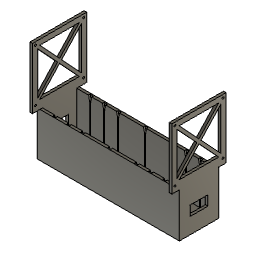
20220624_chipholder (Autodesk Fusion 360 design; units mm, degrees)
Autodesk Fusion 360 part; units mm, degrees
note: some values were not read from the file. Chosen so that the rebuilt part matches the saved one: a direction; which face or edge a step refers to. Set by a fixed rule: which sketch regions a step uses.
sketch "Sketch1" plane through (0, 0, 0) normal (0, 1, 0) x (1, 0, 0)
  line L0 (0, 0) -> (250, 0) construction
  line L1 (0, -70) -> (262.6, -70) construction
  line L2 (0, -80) -> (256.8, -80) construction
  line L3 (25, 0) -> (25, -70)
  line L4 (26.8, -70) -> (26.8, 0)
  line L5 (25, -70) -> (23, -80)
  line L6 (26.8, -70) -> (28.8, -80)
  line L7 (51.8, 0) -> (51.8, -70)
  line L8 (53.6, -70) -> (53.6, 0)
  line L9 (51.8, -70) -> (49.8, -80)
  line L10 (53.6, -70) -> (55.6, -80)
  line L11 (78.6, -70) -> (78.6, 0)
  line L12 (210.8, 0) -> (210.8, -70)
  line L13 (80.4, -70) -> (80.4, 0)
  line L14 (130.4, 0) -> (130.4, -70)
  line L15 (132.2, -70) -> (132.2, 0)
  line L16 (182.2, 0) -> (182.2, -70)
  line L17 (209, -70) -> (209, 0)
  line L18 (237.6, 0) -> (237.6, -70)
  line L19 (235.8, -70) -> (235.8, 0)
  line L20 (184, 0) -> (184, -70)
  line L21 (78.6, -70) -> (76.6, -80)
  line L22 (80.4, -70) -> (82.4, -80)
  line L23 (130.4, -70) -> (128.4, -80)
  line L24 (182.2, -70) -> (180.2, -80)
  line L25 (235.8, -70) -> (233.8, -80)
  line L26 (237.6, -70) -> (239.6, -80)
  line L27 (132.2, -70) -> (134.2, -80)
  line L28 (184, -70) -> (186, -80)
  line L29 (209, -70) -> (207, -80)
  line L30 (210.8, -70) -> (212.8, -80)
  line L31 (0, -80) -> (262.6, -80)
  line L32 (262.6, -80) -> (262.6, 0)
  line L33 (262.6, 0) -> (0, 0)
  line L34 (0, 0) -> (0, -80)
  dimension "d2" = 70
  dimension "d3" = 80
  dimension "d5" = 1.8
  dimension "d6" = 2
  dimension "d7" = 2
  dimension "d8" = 25
  dimension "d9" = 1.8
  dimension "d10" = 2
  dimension "d11" = 2
  dimension "d12" = 25
  dimension "d13" = 1.8
  dimension "d14" = 50
  dimension "d15" = 1.8
  dimension "d16" = 50
  dimension "d17" = 1.8
  dimension "d18" = 25
  dimension "d19" = 1.8
  dimension "d20" = 25
  dimension "d21" = 1.8
  dimension "d22" = 2
  dimension "d23" = 2
  dimension "d24" = 2
  dimension "d25" = 2
  dimension "d26" = 2
  dimension "d27" = 2
  dimension "d28" = 2
  dimension "d29" = 2
  dimension "d30" = 2
  dimension "d31" = 2
  dimension "d32" = 25
  dimension "d33" = 80
  constraint coincident L0.start L33.end
  constraint horizontal L0
  constraint horizontal L1
  constraint parallel L1 L2
  constraint coincident L0 L3.start
  constraint coincident L1 L3.end
  constraint perpendicular L1 L3
  constraint coincident L1 L4.start
  constraint coincident L0 L4.end
  constraint perpendicular L0 L4
  constraint coincident L2 L5.end
  constraint coincident L2 L6.end
  constraint coincident L0 L7.start
  constraint coincident L1 L7.end
  constraint perpendicular L1 L7
  constraint coincident L1 L8.start
  constraint coincident L0 L8.end
  constraint perpendicular L0 L8
  constraint coincident L2 L9.end
  constraint coincident L2 L10.end
  constraint coincident L1 L11.start
  constraint coincident L0 L11.end
  constraint perpendicular L0 L11
  constraint coincident L0 L12.start
  constraint coincident L1 L12.end
  constraint coincident L1 L13.start
  constraint coincident L0 L13.end
  constraint perpendicular L0 L13
  constraint coincident L0 L14.start
  constraint coincident L1 L14.end
  constraint perpendicular L1 L14
  constraint coincident L1 L15.start
  constraint coincident L0 L15.end
  constraint perpendicular L0 L15
  constraint coincident L0 L16.start
  constraint coincident L1 L16.end
  constraint perpendicular L1 L16
  constraint coincident L1 L17.start
  constraint coincident L0 L17.end
  constraint perpendicular L0 L17
  constraint coincident L0 L18.start
  constraint coincident L1 L18.end
  constraint perpendicular L1 L18
  constraint coincident L1 L19.start
  constraint coincident L0 L19.end
  constraint perpendicular L0 L19
  constraint coincident L0 L20.start
  constraint perpendicular L0 L20
  constraint coincident L2 L21.end
  constraint coincident L2 L22.end
  constraint midpoint L2 L23.end
  constraint coincident L2 L24.end
  constraint coincident L2 L25.end
  constraint coincident L2 L26.end
  constraint coincident L1 L20.end
  constraint coincident L2 L27.end
  constraint coincident L2 L28.end
  constraint coincident L2 L29.end
  constraint coincident L2 L30.end
  constraint horizontal L31
  constraint vertical L32
  constraint horizontal L33
  constraint vertical L34
  constraint coincident L1.end L32
  measures "d2" distance of L0 L1
  measures "d3" distance of L0 L2
  measures "d5" distance of L3 L4
  measures "d6" distance of L3 L5.end
  measures "d7" distance of L4 L6.end
  measures "d8" distance of L4 L7
  measures "d9" distance of L7 L8
  measures "d10" distance of L7 L9.end
  measures "d11" distance of L8 L10.end
  measures "d12" distance of L8 L11
  measures "d13" distance of L11 L13
  measures "d14" distance of L13 L14
  measures "d15" distance of L14 L15
  measures "d16" distance of L15 L16
  measures "d17" distance of L16 L20
  measures "d18" distance of L17 L20
  measures "d19" distance of L12 L17
  measures "d20" distance of L12 L19
  measures "d21" distance of L18 L19
  measures "d22" distance of L11 L21.end
  measures "d23" distance of L13 L22.end
  measures "d24" distance of L14 L23.end
  measures "d25" distance of L15 L27.end
  measures "d26" distance of L16 L24.end
  measures "d27" distance of L20 L28.end
  measures "d28" distance of L17 L29.end
  measures "d29" distance of L12 L30.end
  measures "d30" distance of L19 L25.end
  measures "d31" distance of L18 L26.end
  measures "d32" distance of L18 L32
  measures "d33" distance of L31 L33
extrude "Extrude1" add sketch "Sketch1" along normal blind 5 makes body 1
extrude "Extrude2" cut sketch "Sketch1" along normal blind 3 contours L3 L4 L5 L6 L31 L33 | L7 L8 L9 L10 L31 L33 | L11 L13 L21 L22 L31 L33 | L14 L15 L23 L27 L31 L33 | L16 L20 L24 L28 L31 L33 | L12 L17 L29 L30 L31 L33 | L18 L19 L25 L26 L31 L33 bodies 1
copy_body "CopyPasteBodies1" bodies 1 makes body 2
move_body "Move1" bodies 2 to x (1, 0, 0) y (0, 1, 0) z (0, 0, 1) at (0, -71.4, 0)
move_body "Move2" bodies 2 to x (-1, 0, 0) y (0, -1, 0) z (0, 0, 1) at (260.8, -142.8, 0)
move_body "Move3" bodies 2 to x (1, 0, 0) y (0, 1, 0) z (0, 0, 1) at (0, 6, 0)
sketch "Sketch1 (2)" plane through (0, 0, 0) normal (0, 0, 1) x (1, 0, 0) in component "carrier"
  line L0 (-40.0005, -7.3553) -> (29.9995, -7.3553)
  line L1 (29.9995, -7.3553) -> (29.9995, 62.6447)
  line L2 (-40.0005, 62.6447) -> (-40.0005, -7.3553)
  line L3 (-40.0005, 62.6447) -> (-31.0005, 62.6447)
  line L4 (29.9995, 62.6447) -> (20.9995, 62.6447)
  line L5 (-31.0005, 62.6447) -> (-31.0005, 79.6447)
  line L6 (20.9995, 62.6447) -> (20.9995, 79.6447)
  line L7 (20.9995, 79.6447) -> (44.9995, 79.6447)
  line L8 (44.9995, 79.6447) -> (44.9995, 187.4447)
  line L9 (44.9995, 187.4447) -> (-55.0005, 187.4447)
  line L10 (-55.0005, 187.4447) -> (-55.0005, 79.6447)
  line L11 (-55.0005, 79.6447) -> (-31.0005, 79.6447)
  circle A0 centre (-51.1505, 83.4947) radius 1.95
  circle A1 centre (41.1495, 83.4947) radius 1.95
  circle A2 centre (41.1495, 183.5947) radius 1.95
  circle A3 centre (-51.1505, 183.5947) radius 1.95
  line L12 (75.2881, -7.3553) -> (70.2881, -7.3553)
  dimension "d18_1" = 70
  dimension "d23_1" = 9
  dimension "d24_1_1" = 9
  dimension "d25_1_1" = 70
  dimension "d26_1_1" = 52
  dimension "d27_1_1" = 17
  dimension "d28_1" = 17
  dimension "d29_1_1" = 70
  dimension "d47" = 107.8
  dimension "d48" = 100
  dimension "d49" = 3.9
  dimension "d50" = 3.85
  dimension "d51" = 3.85
  dimension "d52" = 3.9
  dimension "d53" = 3.9
  dimension "d54" = 3.9
  dimension "d55" = 3.85
  dimension "d56" = 3.85
  dimension "d57" = 3.85
  dimension "d58" = 3.85
  dimension "d59" = 3.85
  dimension "d60" = 3.85
  constraint horizontal L0
  constraint vertical L1
  constraint vertical L2
  constraint perpendicular L1 L4
  constraint perpendicular L6 L7
  constraint perpendicular L7 L8
  constraint perpendicular L8 L9
  constraint perpendicular L9 L10
  constraint perpendicular L5 L11
  constraint equal L7 L11
  constraint collinear L0 L12
  constraint parallel L0 L9
  measures "d18_1" distance of L0.start L0.end
  measures "d23_1" distance of L2.start L3.end
  measures "d24_1_1" distance of L1.end L4.end
  measures "d25_1_1" distance of L0.end L1.end
  measures "d26_1_1" distance of L5.end L6.end
  measures "d27_1_1" distance of L4.end L6.end
  measures "d28_1" distance of L3.end L5.end
  measures "d29_1_1" distance of L0.start L2.start
  measures "d47" distance of L9 L11
  measures "d48" distance of L8 L10
  measures "d49" diameter of A0
  measures "d50" distance of L11 A0.centre
  measures "d51" distance of L10 A0.centre
  measures "d52" diameter of A1
  measures "d53" diameter of A2
  measures "d54" diameter of A3
  measures "d55" distance of L7 A1.centre
  measures "d56" distance of L8 A1.centre
  measures "d57" distance of L9 A3.centre
  measures "d58" distance of L10 A3.centre
  measures "d59" distance of L9 A2.centre
  measures "d60" distance of L8 A2.centre
extrude "Extrude1'" add sketch "Sketch1 (2)" along normal blind 1.6 separate body contours L0 L1 L2 L3 L4 L5 L6 L7 L8 L9 L10 L11 | A0 | A1 | A2 | A3 makes body 3 in component "carrier"
sketch "Sketch2" plane through (0, 0, 1.7) normal (0, 0, 1) x (-1, 0, 0) in component "carrier"
  line L0 (-200, -70) -> (-200, 0)
  line L1 (-200, 0) -> (-270, 0)
  line L2 (-270, 0) -> (-270, -70)
  line L3 (-270, -70) -> (-261, -70)
  line L4 (-261, -70) -> (-261, -83.4)
  line L5 (-261, -83.4) -> (-209, -83.4)
  line L6 (-209, -83.4) -> (-209, -70)
  line L7 (-209, -70) -> (-200, -70)
  line L8 (-207, -21) -> (-207, -49)
  line L9 (-270, 0) -> (-268.2738, 0)
  line L10 (-268.2738, -21) -> (-270, -21)
  line L11 (-270, -21) -> (-268.2738, -21)
  line L12 (-263, -21) -> (-263, -49)
  line L13 (-207, -49) -> (-263, -49)
  line L14 (-207, -21) -> (-263, -21)
  dimension "d38_1" = 7
  dimension "d39_1_1" = 7
  dimension "d40_1_1" = 21
  dimension "d41_1_1" = 21
  constraint horizontal L9
  constraint horizontal L10
  constraint coincident L1.end L2.start
  constraint perpendicular L2 L11
  constraint perpendicular L11 L12
  measures "d38_1" distance of L0 L8
  measures "d39_1_1" distance of L2 L12
  measures "d40_1_1" distance of L1 L14
  measures "d41_1_1" distance of L3 L13
extrude "Extrude2'" [suppressed] in component "carrier"
sketch "Sketch3" plane through (0, 0, 6.2) normal (0, 0, 1) x (-1, 0, 0) in component "carrier"
  line L0 (-207, -49) -> (-207, -21)
  line L1 (-207, -21) -> (-263, -21)
  line L2 (-263, -21) -> (-263, -49)
  line L3 (-263, -49) -> (-207, -49)
  circle A0 centre (-209.7, -35) radius 2.7
  line L4 (-270, 0) -> (-235, 0) construction
  line L5 (-235, 0) -> (-235, -95) construction
  circle A1 centre (-260.3, -35) radius 2.7
  dimension "d44_1_1" = 5.4
  dimension "d45_1" = 14
  dimension "d47_1" = 2.7
  dimension "d48_1" = 35
  dimension "d49_1" = 14
  dimension "d50_1" = 2.7
  constraint horizontal L4
  constraint perpendicular L1 L5
  constraint symmetric A0 L5 A1
  measures "d44_1_1" diameter of A0
  measures "d45_1" distance of L1 A0.centre
  measures "d47_1" distance of L0 A0.centre
  measures "d48_1" distance of L4.start L4.end
  measures "d49_1" distance of L3 A1.centre
  measures "d50_1" distance of L2 A1.centre
extrude "Extrude4" [suppressed] in component "carrier"
extrude "Extrude3" [suppressed] in component "carrier"
sketch "Sketch5" plane through (0, 0, 0) normal (0, 0, -1) x (1, 0, 0) in component "carrier"
  line L0 (200, 0) -> (200, -70)
  line L1 (200, -70) -> (209, -70)
  line L2 (209, -70) -> (209, -83.4)
  line L3 (209, -83.4) -> (261, -83.4)
  line L4 (261, -83.4) -> (261, -70)
  line L5 (261, -70) -> (270, -70)
  line L6 (270, -70) -> (270, 0)
  line L7 (270, 0) -> (200, 0)
  line L8 (206.7865, -21) -> (206.7865, -49)
  line L9 (263, -21) -> (263, -49)
  line L10 (206.7865, -21) -> (263, -21)
  line L11 (206.7865, -49) -> (263, -49)
  dimension "d61_1" = 28
  dimension "d62_1" = 28
  constraint perpendicular L9 L10
  constraint perpendicular L9 L11
  measures "d61_1" distance of L8.start L8.end
  measures "d62_1" distance of L9.start L9.end
extrude "Extrude6" [suppressed] in component "carrier"
sketch "Sketch7" plane through (0, 0, -4.5) normal (0, 0, -1) x (1, 0, 0) in component "carrier"
  line L0 (206.7865, -21) -> (206.7865, -49)
  line L1 (206.7865, -49) -> (263, -49)
  line L2 (263, -49) -> (263, -21)
  line L3 (263, -21) -> (206.7865, -21)
  circle A0 centre (209.4865, -35) radius 2.7
  line L4 (206.7865, -21) -> (206.7865, -49)
  line L5 (206.7865, -21) -> (263, -21)
  line L6 (235, 0) -> (235, -95)
  circle A1 centre (260.5135, -35) radius 2.7
  dimension "d73_1" = 5.4
  dimension "d74_1" = 2.7
  dimension "d75_1" = 14
  constraint symmetric A0 L6 A1
  measures "d73_1" diameter of A0
  measures "d74_1" distance of A0.centre L4
  measures "d75_1" distance of A0.centre L5
extrude "Extrude8" [suppressed] in component "carrier"
extrude "Extrude7" [suppressed] in component "carrier"
sketch "Sketch8" plane through (0, 0, -6.8) normal (0, 0, -1) x (1, 0, 0) in component "carrier"
  circle A0 centre (209.4865, -35) radius 2.7
  circle A1 centre (209.4865, -35) radius 1.5
  dimension "d80_1" = 3
  constraint concentric A0 A1
  measures "d80_1" diameter of A1
extrude "Extrude9" [suppressed] in component "carrier"
sketch "Sketch10" plane through (0, 0, -6.8) normal (0, 0, -1) x (1, 0, 0) in component "carrier"
  line L0 (263, -36.0522) -> (263, -33.9478)
  arc A0 (263, -33.9478) -> (263, -36.0522) centre (260.5135, -35) ccw
  circle A1 centre (260.5135, -35) radius 1.5
  dimension "d84_1" = 3
  constraint concentric A0 A1
  measures "d84_1" diameter of A1
extrude "Extrude10" [suppressed] in component "carrier"
sketch "Sketch1 (3)" plane through (0, 0, 1.6) normal (0, 0, 1) x (-1, 0, 0) in component "alpide sensor"
  circle A0 centre (-65, -5) radius 1.5
  circle A1 centre (-5, -5) radius 1.5
  circle A2 centre (-65, -65) radius 1.5
  circle A3 centre (-5, -65) radius 1.5
  line L0 (0, -70) -> (0, 0)
  line L1 (0, 0) -> (-70, 0)
  line L2 (-70, 0) -> (-70, -70)
  line L3 (-70, -70) -> (-61, -70)
  line L4 (-61, -70) -> (-61, -83.5)
  line L5 (-61, -83.5) -> (-9, -83.5)
  line L6 (-9, -83.5) -> (-9, -70)
  line L7 (-9, -70) -> (0, -70)
  line L8 (-20, -42.5) -> (-50, -42.5)
  line L9 (-50, -42.5) -> (-50, -27.5)
  line L10 (-50, -27.5) -> (-20, -27.5)
  line L11 (-20, -27.5) -> (-20, -42.5)
  dimension "d58_1" = 30
  dimension "d59_1" = 15
  dimension "d60_1" = 41
  dimension "d63_1" = 20
  constraint horizontal L8
  constraint vertical L9
  constraint horizontal L10
  constraint vertical L11
  measures "d58_1" distance of L8.start L8.end
  measures "d59_1" distance of L8.start L10.end
  measures "d60_1" distance of L5 L8
  measures "d63_1" distance of L2 L9
extrude "Extrude1''" add sketch "Sketch1 (3)" along normal blind -1.8 and the other way blind -0.1 separate body contours L8 L9 L10 L11 makes body 4 in component "alpide sensor"
move_body "Move4" bodies 2 to x (1, 0, 0) y (0, 1, 0) z (0, 0, 1) at (1.7002, -8.1148, 0)
move_body "Move5" bodies 2 to x (1, 0, 0) y (0, 1, 0) z (0, 0, 1) at (0.0998, 78.5148, 0)
move_body "Move6" bodies 2 to x (1, 0, 0) y (0, 1, 0) z (0, 0, 1) at (0, -71.4, 0)
move_body "Move7" bodies 2 to x (1, 0, 0) y (0, 1, 0) z (0, 0, 1) at (0, 1, 0)
sketch "Sketch2 (2)" plane through (0, 0, 0) normal (0, 0, -1) x (1, 0, 0)
  line L0 (182.2, -3) -> (182.2, 0)
  line L1 (182.2, 0) -> (132.2, 0)
  line L2 (132.2, 0) -> (132.2, -3)
  line L3 (132.2, -3) -> (130.4, -3)
  line L4 (130.4, -3) -> (130.4, 0)
  line L5 (130.4, 0) -> (80.4, 0)
  line L6 (80.4, 0) -> (80.4, -3)
  line L7 (80.4, -3) -> (78.6, -3)
  line L8 (78.6, -3) -> (78.6, 0)
  line L9 (78.6, 0) -> (53.6, 0)
  line L10 (53.6, 0) -> (53.6, -3)
  line L11 (53.6, -3) -> (51.8, -3)
  line L12 (51.8, -3) -> (51.8, 0)
  line L13 (51.8, 0) -> (26.8, 0)
  line L14 (26.8, 0) -> (26.8, -3)
  line L15 (26.8, -3) -> (25, -3)
  line L16 (25, -3) -> (25, 0)
  line L17 (25, 0) -> (0, 0)
  line L18 (0, 0) -> (0, -5)
  line L19 (0, -5) -> (262.6, -5)
  line L20 (262.6, -5) -> (262.6, 0)
  line L21 (262.6, 0) -> (237.6, 0)
  line L22 (237.6, 0) -> (237.6, -3)
  line L23 (237.6, -3) -> (235.8, -3)
  line L24 (235.8, -3) -> (235.8, 0)
  line L25 (235.8, 0) -> (210.8, 0)
  line L26 (210.8, 0) -> (210.8, -3)
  line L27 (210.8, -3) -> (209, -3)
  line L28 (209, -3) -> (209, 0)
  line L29 (209, 0) -> (184, 0)
  line L30 (184, 0) -> (184, -3)
  line L31 (184, -3) -> (182.2, -3)
  line L32 (0, 70.4) -> (262.6, 70.4)
  line L33 (262.6, 70.4) -> (262.6, -5)
  line L34 (262.6, -5) -> (0, -5)
  line L35 (0, -5) -> (0, 70.4)
  line L36 (0, 70.4) -> (262.6, 70.4)
  line L37 (262.6, 65.4) -> (262.6, 70.4)
  constraint horizontal L32
  constraint vertical L33
  constraint horizontal L34
  constraint vertical L35
  constraint collinear L32 L36
  constraint collinear L33 L37
  constraint collinear L19 L34
  constraint collinear L18 L35
extrude "Extrude3'" add sketch "Sketch2 (2)" along normal blind 5 separate body makes body 5
extrude "Extrude11" cut sketch "Sketch1 (2)" along normal blind 5 contours A0 | A1 | A2 | A3 bodies 3 in component "carrier"
move_body "Move1'" bodies 3 to x (1, 0, 0) y (0, 1, 0) z (0, 0, 1) at (42.3005, 7.3553, -0.1) in component "carrier"
move_body "Move2'" bodies 3 to x (1, 0, 0) y (0, 1, 0) z (0, 0, 1) at (-3, 0, 0) in component "carrier"
move_body "Move3'" bodies 3 to x (1, 0, 0) y (0, 1, 0) z (0, 0, 1) at (0.7, 0, 0.1) in component "carrier"
sketch "Sketch4" plane through (0, 0, 0) normal (-1, 0, 0) x (0, -1, 0)
  line L0 (0, 0) -> (0, 80)
  line L1 (0, 80) -> (-5, 80)
  line L2 (-5, 80) -> (-5, 0)
  line L3 (-5, 0) -> (0, 0)
  line L4 (-5, 80) -> (0, 80)
  line L5 (70.4, 80) -> (70.4, -5)
  line L6 (70.4, -5) -> (-5, -5)
  line L7 (-5, -5) -> (-5, 80)
  line L8 (70.4, 80) -> (70.4, 0)
  line L9 (70.4, -5) -> (-5, -5)
  line L10 (65.4, 80) -> (70.4, 80)
  line L11 (17.7, 42.5) -> (47.7, 42.5)
  line L12 (47.7, 42.5) -> (47.7, 27.5)
  line L13 (47.7, 27.5) -> (17.7, 27.5)
  line L14 (17.7, 27.5) -> (17.7, 42.5)
  line L15 (17.7, 42.5) -> (17.7, 27.5)
  line L16 (47.7, 42.5) -> (17.7, 42.5)
  line L17 (47.7, 27.5) -> (47.7, 42.5)
  line L18 (17.7, 27.5) -> (47.7, 27.5)
  line L19 (15.7, 44.5) -> (49.7, 44.5)
  line L20 (49.7, 44.5) -> (49.7, 25.5)
  line L21 (49.7, 25.5) -> (15.7, 25.5)
  line L22 (15.7, 25.5) -> (15.7, 44.5)
  line L23 (-19.3, 196.8) -> (84.7, 196.8)
  line L24 (84.7, 196.8) -> (84.7, 80)
  line L25 (-19.3, 80) -> (-19.3, 196.8)
  line L26 (82.7, 194.8) -> (-17.3, 194.8)
  line L27 (82.7, 87) -> (82.7, 194.8)
  line L28 (-17.3, 194.8) -> (-17.3, 87)
  circle A0 centre (78.85, 90.85) radius 1.95
  circle A1 centre (78.85, 90.85) radius 1.95
  circle A2 centre (78.85, 190.95) radius 1.95
  circle A3 centre (78.85, 190.95) radius 1.95
  circle A4 centre (-13.45, 190.95) radius 1.95
  circle A5 centre (-13.45, 190.95) radius 1.95
  circle A6 centre (-13.45, 90.85) radius 1.95
  circle A7 centre (-13.45, 90.85) radius 1.95
  line L29 (84.7, 80) -> (70.4, 80)
  line L30 (0, 80) -> (-19.3, 80)
  line L31 (-9.3, 186.8) -> (74.7, 186.8)
  line L32 (74.7, 186.8) -> (74.7, 96.85)
  line L33 (74.7, 96.85) -> (-9.3, 96.85)
  line L34 (-9.3, 96.85) -> (-9.3, 186.8)
  line L35 (-9.3, 100.85) -> (28.8385, 141.825)
  line L36 (32.7, 145.9737) -> (70.7, 186.8)
  line L37 (74.7, 182.8) -> (36.5615, 141.825)
  line L38 (32.7, 137.6762) -> (-5.3, 96.85)
  line L39 (74.7, 100.85) -> (36.5615, 141.825)
  line L40 (32.7, 145.9737) -> (-5.3, 186.8)
  line L41 (-9.3, 182.8) -> (28.8385, 141.825)
  line L42 (32.7, 137.6762) -> (70.7, 96.85)
  point P0 (-5, 80)
  dimension "d63" = 2
  dimension "d64" = 2
  dimension "d65" = 2
  dimension "d66" = 2
  dimension "d68" = 2
  dimension "d69" = 2
  dimension "d70" = 2
  dimension "d71" = 3.9
  dimension "d72" = 3.9
  dimension "d73" = 3.9
  dimension "d74" = 3.9
  dimension "d75" = 10
  dimension "d76" = 10
  dimension "d77" = 10
  dimension "d78" = 6
  dimension "d79" = 4
  dimension "d80" = 4
  dimension "d81" = 4
  dimension "d82" = 4
  dimension "d83" = 4
  dimension "d84" = 4
  dimension "d85" = 4
  dimension "d86" = 4
  constraint horizontal L4
  constraint vertical L5
  constraint horizontal L6
  constraint vertical L7
  constraint collinear L5 L8
  constraint collinear L6 L9
  constraint collinear L2 L7
  constraint collinear L4 L10
  constraint horizontal L11
  constraint vertical L12
  constraint horizontal L13
  constraint vertical L14
  constraint collinear L14 L15
  constraint collinear L11 L16
  constraint collinear L12 L17
  constraint collinear L13 L18
  constraint horizontal L19
  constraint vertical L20
  constraint horizontal L21
  constraint vertical L22
  constraint horizontal L23
  constraint vertical L24
  constraint horizontal L29
  constraint vertical L25
  constraint coincident P0 L29
  constraint concentric A0 A1
  constraint concentric A2 A3
  constraint concentric A4 A5
  constraint concentric A6 A7
  constraint collinear L29 L30
  constraint horizontal L31
  constraint vertical L32
  constraint horizontal L33
  constraint vertical L34
  constraint coincident L34 L35.start
  constraint coincident L31 L36.end
  constraint coincident L32 L37.start
  constraint coincident L33 L38.end
  constraint coincident L34 L41.start
  constraint coincident L33 L42.end
  constraint coincident L32 L39.start
  constraint coincident L31 L40.end
  constraint coincident L36.start L39
  constraint collinear L35 L36
  constraint coincident L38.start L41
  constraint collinear L37 L38
  constraint collinear L39 L40
  constraint collinear L41 L42
  measures "d63" distance of L11 L19
  measures "d64" distance of L12 L20
  measures "d65" distance of L13 L21
  measures "d66" distance of L14 L22
  measures "d68" distance of L23 L26
  measures "d69" distance of L24 L27
  measures "d70" distance of L25 L28
  measures "d71" diameter of A0
  measures "d72" diameter of A2
  measures "d73" diameter of A4
  measures "d74" diameter of A6
  measures "d75" distance of L25 L34
  measures "d76" distance of L23 L31
  measures "d77" distance of L24 L32
  measures "d78" distance of A6.centre L33
  measures "d79" distance of L33.end L35.start
  measures "d80" distance of L31.end L36.end
  measures "d81" distance of L33.end L38.end
  measures "d82" distance of L31.end L37.start
  measures "d83" distance of L31.start L40.end
  measures "d84" distance of L31.start L41.start
  measures "d85" distance of L32.end L39.start
  measures "d86" distance of L32.end L42.end
extrude "Extrude5" add sketch "Sketch4" along normal blind 5 separate body contours L0 L1 L2 L3 L4 L7 L30 | L0 L1 L3 L4 L5 L6 L7 L8 L9 L23 L24 L25 L29 L30 | L31 L32 L33 L34 L35 L36 L37 L38 L39 L40 L41 L42 makes body 6
copy_body "CopyPasteBodies2" bodies 6 makes body 7
move_body "Move8" bodies 7 to x (1, 0, 0) y (0, 1, 0) z (0, 0, 1) at (267.6, 0, 0)
combine "Combine1" operation add target body 6 tool bodies 1 7 2 5
component "carrier chip v5" placed x (0, -1, 0) y (0, 0, 1) z (-1, 0, 0) at (45.4, 73.6, 4.0098)
component "carrier" placed x (1, 0, 0) y (0, 1, 0) z (0, 0, 1) at (71.3, -4.0098, 18.7) in component "carrier chip v5"
component "alpide sensor" placed x (1, 0, 0) y (0, 1, 0) z (0, 0, 1) at (0, 0, 0) in component "carrier"
equation "d4 = 25 mm"
equation "d7 = d6"
equation "d8 = d4"
equation "d9 = d5"
equation "d10 = d6"
equation "d11 = d6"
equation "d12 = d4"
equation "d13 = d5"
equation "d15 = d5"
equation "d16 = d14"
equation "d17 = d5"
equation "d18 = d4"
equation "d19 = d5"
equation "d20 = d4"
equation "d21 = d5"
equation "d22 = d6"
equation "d23 = d6"
equation "d24 = d6"
equation "d25 = d6"
equation "d26 = d6"
equation "d27 = d6"
equation "d28 = d6"
equation "d29 = d6"
equation "d30 = d6"
equation "d31 = d6"
equation "d32 = d4"
equation "d27_1_1 = d28_1"
equation "d50 = 1.9 mm + ( 3.9 / 2 ) * 1 mm"
equation "d51 = 1.9 mm + ( 3.9 / 2 ) * 1 mm"
equation "d55 = d50"
equation "d56 = d51"
equation "d57 = d50"
equation "d58 = d51"
equation "d59 = d57"
equation "d60 = d58"
equation "d76 = d75"
equation "d77 = d76"
equation "d78 = 4 mm + 2 mm"
equation "d81 = d79"
equation "d86 = d85"
